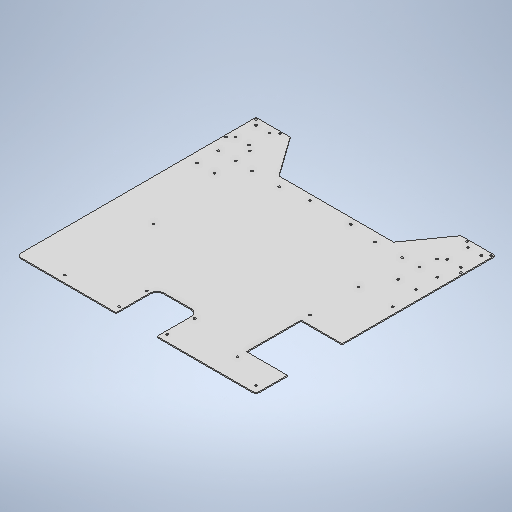
# Autodesk Inventor part: 知能ロボ土台
Saved by Autodesk Inventor 2026.2 (Build 302298010, 298A)
## iProperties
Created: 2026-04-20
Part Number: 知能ロボ土台
Material: Generic
Document SubType Name: Modeling
Designer: Yagis
Density: 1 g/cm^3
Appearance: Default
Author: Yagis
Autodesk Inventor part; units mm, degrees
ref_plane "YZ Plane" through (0, 0, 0) normal (1, 0, 0) x (0, 1, 0)
ref_plane "XZ Plane" through (0, 0, 0) normal (0, 1, 0) x (-1, 0, 0)
ref_plane "XY Plane" through (0, 0, 0) normal (0, 0, 1) x (1, 0, 0)
sketch "スケッチ1" plane through (0, 0, 0) normal (0, 1, 0) x (-1, 0, 0)
  line L0 (-170, 175) -> (170, 175)
  line L1 (175, 170) -> (175, -122)
  line L2 (165, -175) -> (-165, -175)
  line L3 (-175, -165) -> (-175, 170)
  arc A0 (175, 170) -> (170, 175) centre (170, 170) ccw
  arc A1 (-170, 175) -> (-175, 170) centre (-170, 170) ccw
  circle A2 centre (0, -266.9818) radius 37.5
  line L4 (175, -111) -> (99.9, -111)
  line L5 (99.9, -111) -> (99.9, -76)
  line L6 (99.9, -76) -> (175, -76)
  line L7 (175, -76) -> (175, -111)
  line L8 (-99.9, -111) -> (-175, -111)
  line L9 (-175, -111) -> (-175, -76)
  line L10 (-175, -76) -> (-99.9, -76)
  line L11 (-99.9, -76) -> (-99.9, -111)
  line L12 (-165, -165) -> (-99.9, -111)
  line L13 (165, -165) -> (99.9, -111)
  line L14 (-175, 145.8165) -> (0, 145.8165)
  line L15 (0, 145.8165) -> (99.9, -76)
  line L16 (-175, 54.0733) -> (-99.9, 54.0733)
  line L17 (-99.9, 54.0733) -> (-99.9, -76)
  line L18 (142.7273, 44.6356) -> (87.7273, 44.6356)
  line L19 (87.7273, 44.6356) -> (87.7273, 114.6356)
  line L20 (87.7273, 114.6356) -> (142.7273, 114.6356)
  line L21 (142.7273, 114.6356) -> (142.7273, 44.6356)
  line L22 (-175, -165) -> (-175, -174)
  line L23 (-165, -175) -> (-174, -175)
  line L24 (174, -175) -> (165, -175)
  line L25 (175, -175) -> (175, -175)
  line L26 (175, -122) -> (175, -174)
  line L27 (0, -175) -> (0, -111)
  line L28 (-175, -175) -> (-175, -175)
  arc A3 (174, -175) -> (175, -174) centre (174, -174) ccw
  arc A4 (-175, -174) -> (-174, -175) centre (-174, -174) ccw
  point P0 (0, 0)
  point P1 (175, 175)
  point P2 (172.5, -105)
  point P3 (172.5, -81)
  point P4 (-172.5, -105)
  point P5 (-172.5, -81)
  point P6 (-99.9, -93.5)
  point P7 (99.9, -93.5)
  point P8 (-30, -155)
  point P9 (30, -155)
  dimension "d0" = 350
  dimension "d1" = 350
  dimension "d2" = 175
  dimension "d3" = 175
  dimension "d4" = 5
  dimension "d5" = 75
  dimension "d17" = 75.1
  dimension "d18" = 35
  dimension "d19" = 75.1
  dimension "d20" = 35
  dimension "d21" = 24
  dimension "d22" = 6
  dimension "d23" = 2.5
  dimension "d24" = 6
  dimension "d25" = 24
  dimension "d26" = 2.5
  dimension "d27" = 70
  dimension "d44" = 60
  dimension "d45" = 30
  dimension "d46" = 20
  dimension "d47" = 55
  dimension "d48" = 70
  dimension "d107" = 1
  dimension "d108" = 1
  constraints: 58 end point, 15 point on line, 8 parallel, 8 point on circle, 8 tangent, 7 horizontal, 6 perpendicular, 5 centre point, 3 midpoint, 2 horizontal alignment, 2 vertical, 2 vertical alignment, 1 collinear, 1 equal radius, 1 symmetric about line
  measures "d0" distance of point (175, 175) L25.start
  measures "d1" distance of L25.start L28.start
  measures "d2" distance from line of L2 point (0, 0)
  measures "d3" distance from line of point (0, 0) L1
  measures "d4" radius of A0
  measures "d5" diameter of A2
  measures "d17" distance of L4.start L4.end
  measures "d18" distance of L4.end L5.end
  measures "d19" distance of L8.start L9.start
  measures "d20" distance of L9.start L9.end
  measures "d21" distance of point (172.5, -81) point (172.5, -105)
  measures "d22" distance from line of L4 point (172.5, -105)
  measures "d23" distance from line of L7 point (172.5, -105)
  measures "d24" distance from line of L8 point (-172.5, -105)
  measures "d25" distance of point (-172.5, -81) point (-172.5, -105)
  measures "d26" distance from line of L3 point (-172.5, -105)
  measures "d27" distance from line of point (172.5, -105) L2
  measures "d44" distance of point (30, -155) point (-30, -155)
  measures "d45" horizontal distance of point (30, -155) L27.start
  measures "d46" distance from line of L2 point (-30, -155)
  measures "d47" distance of L19.end L20.end
  measures "d48" distance of L18.end L19.end
  measures "d107" radius of A3
  measures "d108" radius of A4
extrude "押し出し1" add sketch "スケッチ1" along normal blind 1.5 contours L0 A0 L1 L6 L15 L14 L3 A1 | L14 L15 L5 L4 L1 L26 A3 L24 L2 L23 A4 L22 L3 L8 L11 L17 L16 | L1 L4 L5 L6 | L16 L17 L10 L3 | L10 L11 L8 L3 | L18 L19 L20 L21
sketch "スケッチ3" plane through (0, 1.5, 0) normal (0, 1, 0) x (1, 0, 0)
  line L0 (-175, 174) -> (-175, -170) projected
  line L1 (175, -170) -> (175, 174) projected
  line L2 (0, 175) -> (0, 0)
  line L3 (165, 175) -> (-165, 175)
  arc A0 (-174, 175) -> (-175, 174) centre (-174, 174) ccw projected
  point P0 (-160.2, 105)
  point P1 (-160.2, 73.8)
  point P2 (160.2, 105)
  point P3 (160.2, 73.8)
  point P4 (-134.6, 105)
  point P5 (-134.6, 73.8)
  point P6 (134.6, 73.8)
  point P7 (134.6, 105)
  point P8 (-30, 109)
  point P9 (30, 109)
  point P10 (-70, 104)
  point P11 (70, 104)
  point P12 (-110, 104)
  point P13 (110, 104)
  point P14 (-137, 172)
  point P15 (-172, 172)
  point P16 (-172, 128)
  point P17 (-137, 128)
  point P18 (137, 172)
  point P19 (172, 172)
  point P20 (172, 128)
  point P21 (137, 128)
  point P22 (-174.7071, 174.7071)
  point P23 (-165, 165)
  point P24 (-165, 135)
  point P25 (-145, 135)
  point P26 (-145, 165)
  point P27 (165, 165)
  point P28 (165, 135)
  point P29 (145, 135)
  point P30 (145, 165)
  dimension "d29" = 31.2
  dimension "d30" = 14.8
  dimension "d31" = 14.8
  dimension "d39" = 25.6
  dimension "d40" = 25.6
  dimension "d41" = 60
  dimension "d42" = 30
  dimension "d75" = 140
  dimension "d76" = 40
  dimension "d77" = 40
  dimension "d78" = 70
  dimension "d94" = 44
  dimension "d95" = 35
  dimension "d104" = 3
  dimension "d110" = 3
  dimension "d118" = 66
  dimension "d122" = 71
  dimension "d123" = 70
  dimension "d130" = 10
  dimension "d131" = 20
  dimension "d132" = 10
  dimension "d133" = 30
  constraints: 14 horizontal alignment, 8 symmetric about line, 8 vertical alignment, 4 end point, 1 horizontal, 1 point on circle, 1 vertical
  measures "d29" distance of point (-160.2, 105) point (-160.2, 73.8)
  measures "d30" distance from line of L0 point (-160.2, 105)
  measures "d31" distance from line of point (160.2, 105) L1
  measures "d39" distance of point (-134.6, 105) point (-160.2, 105)
  measures "d40" distance of point (134.6, 105) point (160.2, 105)
  measures "d41" distance of point (-30, 109) point (30, 109)
  measures "d42" horizontal distance of point (-30, 109) point (0, 175)
  measures "d75" distance of point (-70, 104) point (70, 104)
  measures "d76" distance of point (110, 104) point (70, 104)
  measures "d77" distance of point (-110, 104) point (-70, 104)
  measures "d78" horizontal distance of L2.start point (70, 104)
  measures "d94" distance of point (-172, 172) point (-172, 128)
  measures "d95" distance of point (-137, 172) point (-172, 172)
  measures "d104" distance from line of point (-172, 172) L3
  measures "d110" distance from line of L0 point (-172, 172)
  measures "d118" distance from line of L3 point (-30, 109)
  measures "d122" distance from line of L3 point (-110, 104)
  measures "d123" distance from line of L3 point (-160.2, 105)
  measures "d130" distance from line of point (-165, 165) L0
  measures "d131" distance of point (-145, 165) point (-165, 165)
  measures "d132" distance from line of L3 point (-165, 165)
  measures "d133" distance of point (-165, 135) point (-165, 165)
hole "穴2" at (-160.2, 1.5, -105) at (-160.2, 1.5, -73.8) at (160.2, 1.5, -105) at (160.2, 1.5, -73.8) at (-134.6, 1.5, -105) at (-134.6, 1.5, -73.8) at (134.6, 1.5, -73.8) at (134.6, 1.5, -105) at (-30, 1.5, -109) at (30, 1.5, -109) at (-70, 1.5, -104) at (70, 1.5, -104) at (110, 1.5, -104) at (-110, 1.5, -104) at (-172, 1.5, -128) at (-137, 1.5, -128) at (-137, 1.5, -172) at (-172, 1.5, -172) at (137, 1.5, -128) at (172, 1.5, -128) at (172, 1.5, -172) at (137, 1.5, -172) at (-165, 1.5, -165) at (-145, 1.5, -165) at (-145, 1.5, -135) at (-165, 1.5, -135) at (145, 1.5, -165) at (165, 1.5, -165) at (165, 1.5, -135) at (145, 1.5, -135) direction (0, -1, 0) diameter 3.2 depth 10 tip angle 118
sketch "スケッチ4" plane through (0, 1.5, 0) normal (0, 1, 0) x (1, 0, 0)
  line L0 (40, -175) -> (-40, -175)
  line L1 (-40, -175) -> (-40, -115)
  line L2 (-40, -115) -> (40, -115)
  line L3 (40, -115) -> (40, -175)
  line L4 (-170, -175) -> (170, -175) projected
  line L5 (30.0906, -175) -> (-29.9094, -175)
  line L6 (-29.9094, -175) -> (-29.9094, -125)
  line L7 (-19.9094, -115) -> (20.0906, -115)
  line L8 (30.0906, -125) -> (30.0906, -175)
  line L9 (175, -170) -> (175, 174) projected
  line L10 (-175, 174) -> (-175, -170) projected
  arc A0 (-19.9094, -115) -> (-29.9094, -125) centre (-19.9094, -125) ccw
  arc A1 (30.0906, -125) -> (20.0906, -115) centre (20.0906, -125) ccw
  line L11 (175, -129) -> (115, -129)
  line L12 (175, -49) -> (115, -49)
  line L13 (115, -49) -> (115, -129)
  point P0 (0, 0)
  point P1 (-40, -145)
  point P2 (0, -175)
  point P3 (0, -175)
  point P4 (35, -165)
  point P5 (35, -125)
  point P6 (-35, -125)
  point P7 (-35, -165)
  point P8 (-29.9094, -115)
  point P9 (30.0906, -115)
  point P10 (-29.9094, -175)
  point P11 (-115, -165)
  point P12 (165, -165)
  point P13 (165, 35)
  point P14 (-115, -35)
  point P15 (-29.9094, -175)
  point P16 (115, 35)
  point P17 (145, -129)
  point P18 (115, -142)
  point P19 (115, -36)
  dimension "d53" = 60
  dimension "d54" = 80
  dimension "d56" = 0
  dimension "d57" = 5
  dimension "d58" = 5
  dimension "d59" = 40
  dimension "d60" = 10
  dimension "d68" = 60
  dimension "d111" = 10
  dimension "d113" = 200
  dimension "d114" = 280
  dimension "d117" = 10
  dimension "d120" = 130
  dimension "d121" = 50
  dimension "d124" = 46
  dimension "d125" = 80
  dimension "d126" = 60
  dimension "d127" = 13
  dimension "d128" = 13
  dimension "d129" = 60
  constraints: 22 end point, 6 point on line, 5 vertical alignment, 4 midpoint, 4 parallel, 4 point on circle, 4 tangent, 3 horizontal, 3 horizontal alignment, 3 perpendicular, 2 centre point, 1 equal radius, 1 vertical
  measures "d53" distance of L2.end L0.start
  measures "d54" distance from line of point (-40, -145) L3
  measures "d56" distance of point (0, -175) point (0, -175)
  measures "d57" distance from line of L3 point (35, -165)
  measures "d58" distance from line of L1 point (-35, -165)
  measures "d59" distance of point (-35, -125) point (-35, -165)
  measures "d60" distance from line of L0 point (-35, -165)
  measures "d68" distance between parallel lines of L6 L8
  measures "d111" distance from line of L9 point (165, -165)
  measures "d113" distance of point (165, 35) point (165, -165)
  measures "d114" distance of point (165, -165) point (-115, -165)
  measures "d117" radius of A0
  measures "d120" distance of point (-115, -35) point (-115, -165)
  measures "d121" distance of point (165, 35) point (115, 35)
  measures "d124" distance from line of L4 point (145, -129)
  measures "d125" distance between parallel lines of L11 L12
  measures "d126" distance of L12.start L12.end
  measures "d127" distance from line of point (115, -142) L11
  measures "d128" distance from line of point (115, -36) L12
  measures "d129" distance from line of L9 point (115, -142)
hole "穴3" at (35, 1.5, 165) at (35, 1.5, 125) at (-35, 1.5, 125) at (-35, 1.5, 165) at (-115, 1.5, 165) at (-115, 1.5, 35) at (165, 1.5, -35) at (165, 1.5, 165) at (115, 1.5, -35) at (115, 1.5, 36) at (115, 1.5, 142) direction (0, -1, 0) diameter 3.2 depth 8.8 tip angle 118
extrude "押し出し2" cut sketch "スケッチ4" against normal blind 10 contours L0 L6 A0 L2 A1 L8 | L11 L13 L12 L9
sketch "スケッチ5" plane through (0, 1.5, 0) normal (0, 1, 0) x (1, 0, 0)
  line L0 (125, 175) -> (85, 119)
  line L1 (85, 119) -> (-85, 119)
  line L2 (-85, 119) -> (-125, 175)
  line L3 (-175, 174) -> (-175, -170) projected
  line L4 (125, 175) -> (-125, 175)
  line L5 (174, 175) -> (-174, 175) projected
  point P0 (0, 0)
  point P1 (165, 175)
  point P2 (0, 175)
  point P3 (0, 175)
  point P4 (0, 119)
  point P5 (0, 175)
  point P6 (0, 175)
  dimension "d85" = 125
  dimension "d91" = 250
  dimension "d99" = 56
  dimension "d106" = 170
  constraints: 8 end point, 3 vertical alignment, 2 midpoint, 1 horizontal, 1 parallel, 2 other
  measures "d85" distance of point (0, 175) L2.end
  measures "d91" distance of L0.start L2.end
  measures "d99" distance between parallel lines of L4 L1
  measures "d106" distance of L0.end L1.end
extrude "押し出し3" cut sketch "スケッチ5" against normal blind 10
fillet "面フィレット5" radius 1.5 1 edges at (0, 1.5, -119)
